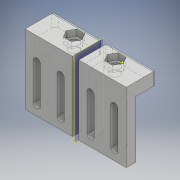
# Autodesk Inventor part: CarroXY - Batente frontal
Saved by Autodesk Inventor 2017 (Build 210142000, 142)
## iProperties
Created: 2020-08-15
Part Number: CarroXY - Batente frontal
Material: Generic
Document SubType Name: Modeling
Designer: ale
Density: 1 g/cm^3
Appearance: Default
Author: ale
Autodesk Inventor part; units mm, degrees
ref_plane "YZ Plane" through (0, 0, 0) normal (1, 0, 0) x (0, 1, 0)
ref_plane "XZ Plane" through (0, 0, 0) normal (0, 1, 0) x (-1, 0, 0)
ref_plane "XY Plane" through (0, 0, 0) normal (0, 0, 1) x (1, 0, 0)
sketch "Sketch1" plane through (0, 0, 0) normal (0, 0, 1) x (1, 0, 0)
  line L0 (-15, 6.5) -> (15, 6.5)
  line L1 (15, 6.5) -> (15, -6.5)
  line L2 (15, -6.5) -> (-15, -6.5)
  line L3 (-15, -6.5) -> (-15, 6.5)
  line L4 (-15, 6.5) -> (15, -6.5) construction
  line L5 (15, 6.5) -> (-15, -6.5) construction
  point P0 (0, 0)
  dimension "d0" = 30
  dimension "d1" = 13
  constraints: 12 end point, 2 midpoint, 2 parallel, 1 horizontal, 1 perpendicular
  measures "d0" distance of L1.end L2.end
  measures "d1" distance of L0.end L1.end
extrude "Extrusion1" add sketch "Sketch1" along normal blind 8
sketch "Sketch2" plane through (-15, -6.5, 0) normal (0, -1, 0) x (1, 0, 0)
  line L0 (0, 0) -> (0, 8) projected
  line L1 (0, 8) -> (30, 8)
  line L2 (30, 8) -> (30, -36)
  line L3 (30, -36) -> (0, -36)
  line L4 (0, -36) -> (0, 8)
  point P0 (15, 0)
  dimension "d4" = 30
  dimension "d5" = 44
  constraints: 8 end point, 2 parallel, 1 horizontal, 1 perpendicular
  measures "d4" distance of L2.end L3.end
  measures "d5" distance of L1.end L2.end
extrude "Extrusion2" add sketch "Sketch2" along normal blind 6
sketch "Sketch3" plane through (0, 0, 8) normal (0, 0, 1) x (1, 0, 0)
  circle A0 centre (-4, -0.5) radius 10
  line L0 (-15, 6.5) -> (-15, -12.5) projected
  line L1 (15, -12.5) -> (-15, -12.5) projected
  point P0 (0, 0)
  dimension "d8" = 20
  dimension "d9" = 11
  dimension "d10" = 12
  constraints: 1 centre point
  measures "d8" diameter of A0
  measures "d9" distance from line of A0.centre L0
  measures "d10" distance from line of A0.centre L1
hole "Hole1" at (-4, -0.5, 8) direction (0, 0, -1) diameter 5.7 end through all
sketch "Sketch4" plane through (0, 0, 8) normal (0, 0, 1) x (1, 0, 0)
  circle A0 centre (-4, -0.5) radius 2.85 projected
  line L0 (-6.4669, 3.8491) -> (-1.467, 3.8109)
  line L1 (-1.467, 3.8109) -> (0.9999, -0.5382)
  line L2 (0.9999, -0.5382) -> (-1.5331, -4.8491)
  line L3 (-1.5331, -4.8491) -> (-6.533, -4.8109)
  line L4 (-6.533, -4.8109) -> (-8.9999, -0.4618)
  line L5 (-8.9999, -0.4618) -> (-6.4669, 3.8491)
  point P0 (0, 0)
  dimension "d18" = 10
  constraints: 12 end point, 1 coincident, 13 other
  measures "d18" distance of L0.end L3.end
sketch "Sketch5" plane through (0, 0, 8) normal (0, 0, 1) x (1, 0, 0)
  point P0 (0, 0)
extrude "Extrusion3" cut sketch "Sketch4" against normal blind 4
sketch "Sketch6" plane through (-15, -6.5, 0) normal (0, 1, 0) x (1, 0, 0)
  arc A0 (24.75, 29.6235) -> (20.25, 29.6235) centre (22.5, 29.6235) ccw
  line L0 (30, 0) -> (30, 36) projected
  line L1 (30, 18) -> (0, 18)
  line L2 (0, -8) -> (0, 36) projected
  line L3 (15, 0) -> (15, 36)
  line L4 (30, 36) -> (0, 36) projected
  arc A1 (20.25, 6.3765) -> (24.75, 6.3765) centre (22.5, 6.3765) ccw
  line L5 (24.75, 6.3765) -> (24.75, 29.6235)
  line L6 (20.25, 6.3765) -> (20.25, 29.6235)
  arc A2 (9.75, 29.6235) -> (5.25, 29.6235) centre (7.5, 29.6235) ccw
  arc A3 (5.25, 6.3765) -> (9.75, 6.3765) centre (7.5, 6.3765) ccw
  line L7 (5.25, 6.3765) -> (5.25, 29.6235)
  line L8 (9.75, 6.3765) -> (9.75, 29.6235)
  dimension "d21" = 4.5
  dimension "d22" = 7.5
  constraints: 12 end point, 8 point on circle, 7 symmetric about line, 4 centre point, 3 tangent, 2 midpoint, 1 horizontal, 1 point on line, 1 vertical, 3 other
  measures "d21" diameter of A0
  measures "d22" distance from line of L0 A0.centre
extrude "Extrusion4" cut sketch "Sketch6" against normal through all contours L5 L1 L6 A0 | L5 A1 L6 L1 | L8 A3 L7 L1 | L1 L7 A2 L8
fillet "Fillet1" radius 2 3 edges at (15, 6.5, 4) (0, 6.5, 8) (-15, 6.5, 4)
ref_plane "Work Plane1" through (-17, -6.5, -36) normal (-1, 0, 0) x (0, 0, 1)
mirror "Mirror1" about plane through (-17, -6.5, -36) normal (-1, 0, 0)
body "Solid1"
